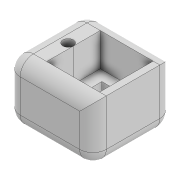
# Autodesk Inventor part: Cable_tie_connector_p1
Saved by Autodesk Inventor 2022 (Build 260153000, 153)
## iProperties
Created: 2022-07-19
Part Number: Cable_tie_connector_p1
Material: Generic
Document SubType Name: Modeling
Designer: dell
Density: 1 g/cm^3
Appearance: Default
Author: dell
Autodesk Inventor part; units mm, degrees
ref_plane "YZ Plane" through (0, 0, 0) normal (1, 0, 0) x (0, 1, 0)
ref_plane "XZ Plane" through (0, 0, 0) normal (0, 1, 0) x (-1, 0, 0)
ref_plane "XY Plane" through (0, 0, 0) normal (0, 0, 1) x (1, 0, 0)
sketch "Sketch1" plane through (0, 0, 0) normal (0, 1, 0) x (-1, 0, 0)
  line L0 (-4, 4.05) -> (4, 4.05)
  line L1 (4, 4.05) -> (4, -4.05)
  line L2 (4, -4.05) -> (-4, -4.05)
  line L3 (-4, -4.05) -> (-4, 4.05)
  line L4 (-4, 4.05) -> (4, -4.05) construction
  line L5 (4, 4.05) -> (-4, -4.05) construction
  line L6 (8, 6.05) -> (-5, 6.05)
  line L7 (-5, 6.05) -> (-5, -6.05)
  line L8 (-5, -6.05) -> (8, -6.05)
  line L9 (8, -6.05) -> (8, 6.05)
  point P0 (0, 0)
  dimension "d0" = 8.1
  dimension "d1" = 8
  dimension "d5" = 2
  dimension "d6" = 2
  dimension "d7" = 1
  dimension "d8" = 4
  constraints: 20 end point, 4 perpendicular, 2 horizontal, 2 midpoint, 2 parallel
  measures "d0" distance of L2.end L0.start
  measures "d1" distance of L1.end L2.end
  measures "d5" distance between parallel lines of L6 L0
  measures "d6" distance between parallel lines of L8 L2
  measures "d7" distance between parallel lines of L3 L7
  measures "d8" distance between parallel lines of L1 L9
extrude "Extrusion1" add sketch "Sketch1" along normal blind 5
sketch "Sketch2" plane through (0, 0, 0) normal (0, -1, 0) x (1, 0, 0)
  line L0 (5, 6.05) -> (5, -6.05) projected
  line L1 (-8, 6.05) -> (5, 6.05) projected
  line L2 (-8, -6.05) -> (-8, 6.05) projected
  line L3 (5, -6.05) -> (-8, -6.05) projected
  line L4 (4, 4.05) -> (-4, 4.05) projected
  line L5 (4, -4.05) -> (4, 4.05) projected
  line L6 (-4, -4.05) -> (4, -4.05) projected
  line L7 (-4, 4.05) -> (-4, -4.05) projected
  point P0 (0, 0)
extrude "Extrusion2" add sketch "Sketch2" along normal blind 4 contours L0 L3 L2 L1 | L5 L6 L7 L4
sketch "Sketch3" plane through (0, 5, 0) normal (0, 1, 0) x (1, 0, 0)
  line L0 (-4, -4.05) -> (-4, 4.05) projected
  circle A0 centre (-4.8, 0) radius 0.8
  point P0 (0, 0)
  dimension "d14" = 1.6
  constraints: 1 centre point, 1 tangent
  measures "d14" diameter of A0
extrude "Extrusion3" cut sketch "Sketch3" against normal blind 100
sketch "Sketch4" plane through (0, 0, 0) normal (0, 1, 0) x (1, 0, 0)
  line L0 (-0.2, -2.5) -> (-2.2, -2.5)
  line L1 (-2.2, -2.5) -> (-2.2, 2.5)
  line L2 (-2.2, 2.5) -> (-0.2, 2.5)
  line L3 (-0.2, 2.5) -> (-0.2, -2.5)
  line L4 (-0.2, -2.5) -> (-2.2, 2.5) construction
  line L5 (-2.2, -2.5) -> (-0.2, 2.5) construction
  line L6 (-4, -4.05) -> (-4, 0) projected
  point P0 (0, 0)
  point P1 (-1.2, 0)
  point P2 (-1.2, 0)
  dimension "d17" = 5
  dimension "d18" = 3.8
  dimension "d19" = 2
  constraints: 12 end point, 3 midpoint, 2 parallel, 1 horizontal, 1 horizontal alignment, 1 perpendicular
  measures "d17" distance of L2.end L0.start
  measures "d18" distance between parallel lines of L6 L3
  measures "d19" distance between parallel lines of L3 L1
extrude "Extrusion4" cut sketch "Sketch4" against normal blind 100
fillet "Fillet1" radius 2 11 edges at (-8, 0.5, -6.05) (5, 0.5, -6.05) (-8, 0.5, 6.05) (5, 0.5, 6.05) (-1.5, -4, 6.05) (-8, -4, 0) (-1.5, -4, -6.05) (-1.5, 5, 6.05) (-8, 5, 0) (-1.5, 5, -6.05) (5, -4, 0)
body "Solid1"
